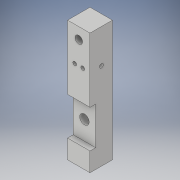
# Autodesk Inventor part: Main Block
Saved by Autodesk Inventor 2018 (Build 220112000, 112)
## iProperties
Created: 2017-09-20
Part Number: Main Block
Material: Generic
Document SubType Name: Modeling
Designer: Intel
Density: 1 g/cm^3
Appearance: Default
Author: Intel
Autodesk Inventor part; units mm, degrees
ref_plane "YZ Plane" through (0, 0, 0) normal (1, 0, 0) x (0, 1, 0)
ref_plane "XZ Plane" through (0, 0, 0) normal (0, 1, 0) x (-1, 0, 0)
ref_plane "XY Plane" through (0, 0, 0) normal (0, 0, 1) x (1, 0, 0)
sketch "Sketch1" plane through (0, 0, 0) normal (0, 0, 1) x (1, 0, 0)
  line L0 (-9.398, 50.8) -> (9.398, 50.8)
  line L1 (9.398, 50.8) -> (9.398, -50.8)
  line L2 (9.398, -50.8) -> (-9.398, -50.8)
  line L3 (-9.398, -50.8) -> (-9.398, 50.8)
  line L4 (-9.398, 50.8) -> (9.398, -50.8) construction
  line L5 (9.398, 50.8) -> (-9.398, -50.8) construction
  point P0 (0, 0)
  dimension "d0" = 18.796
  dimension "d1" = 101.6
  constraints: 12 end point, 2 midpoint, 2 parallel, 1 horizontal, 1 perpendicular
  measures "d0" distance of L1.end L2.end
  measures "d1" distance of L0.end L1.end
extrude "Extrusion1" add sketch "Sketch1" along normal mid plane 18.796
sketch "Sketch2" plane through (0, 0, 9.398) normal (0, 0, 1) x (1, 0, 0)
  line L0 (9.398, -50.8) -> (9.398, 50.8) projected
  line L1 (-9.398, -34.925) -> (9.398, -34.925)
  line L2 (9.398, -34.925) -> (9.398, -3.175)
  line L3 (9.398, -3.175) -> (-9.398, -3.175)
  line L4 (-9.398, -3.175) -> (-9.398, -34.925)
  line L5 (-9.398, -34.925) -> (9.398, -3.175) construction
  line L6 (9.398, -34.925) -> (-9.398, -3.175) construction
  line L7 (-9.398, -50.8) -> (9.398, -50.8) projected
  point P0 (0, 0)
  point P1 (0, -19.05)
  dimension "d4" = 31.75
  dimension "d5" = 15.875
  dimension "d6" = 18.796
  constraints: 12 end point, 2 midpoint, 2 parallel, 1 horizontal, 1 perpendicular, 1 point on line
  measures "d4" distance of L2.end L1.end
  measures "d5" distance between parallel lines of L7 L1
  measures "d6" distance of L2.end L3.end
extrude "Extrusion3" cut sketch "Sketch2" against normal blind 4.7498
sketch "Sketch3" plane through (0, 0, 4.6482) normal (0, 0, 1) x (1, 0, 0)
  circle A0 centre (0, -19.05) radius 3.9624
  line L0 (9.398, -34.925) -> (-9.398, -34.925) projected
  line L1 (9.398, -3.175) -> (9.398, -34.925) projected
  point P0 (0, 0)
  dimension "d11" = 7.9248
  dimension "d12" = 15.875
  dimension "d13" = 9.398
  constraints: 1 centre point
  measures "d11" diameter of A0
  measures "d12" distance from line of L0 A0.centre
  measures "d13" distance from line of L1 A0.centre
extrude "Extrusion4" cut sketch "Sketch3" against normal blind 15.24
sketch "Sketch4" plane through (0, 0, 9.398) normal (0, 0, 1) x (1, 0, 0)
  circle A0 centre (0, 41.275) radius 3.175
  line L0 (9.398, 50.8) -> (-9.398, 50.8) projected
  line L1 (9.398, -3.175) -> (9.398, 50.8) projected
  point P0 (0, 0)
  dimension "d16" = 6.35
  dimension "d17" = 9.525
  dimension "d18" = 9.398
  constraints: 1 centre point
  measures "d16" diameter of A0
  measures "d17" distance from line of L0 A0.centre
  measures "d18" distance from line of L1 A0.centre
extrude "Extrusion5" cut sketch "Sketch4" against normal blind 20.32
sketch "Sketch5" plane through (0, 0, 9.398) normal (0, 0, 1) x (1, 0, 0)
  circle A0 centre (-3.359, 22.225) radius 1.5875
  circle A1 centre (3.359, 22.225) radius 1.5875
  line L0 (9.398, 50.8) -> (-9.398, 50.8) projected
  line L1 (-9.398, 50.8) -> (9.398, 50.8) projected
  line L2 (0, 50.8) -> (0, -50.8) construction
  line L3 (9.398, -50.8) -> (-9.398, -50.8) projected
  circle A2 centre (0, 41.275) radius 3.175 projected
  line L4 (0, 41.275) -> (3.359, 22.225) construction
  line L5 (0, 41.275) -> (-3.359, 22.225) construction
  point P0 (0, 0)
  dimension "d21" = 3.175
  dimension "d22" = 3.175
  dimension "d23" = 28.575
  dimension "d24" = 28.575
  dimension "d25" = 10
  dimension "d26" = 10
  constraints: 6 end point, 2 centre point, 2 midpoint
  measures "d21" diameter of A0
  measures "d22" diameter of A1
  measures "d23" distance from line of L4.end L0
  measures "d24" distance from line of L0 L5.end
  measures "d25" angle of L2 L4
  measures "d26" angle of L5 L2
extrude "Extrusion6" cut sketch "Sketch5" against normal blind 20.32 contours A0
sketch "Sketch6" plane through (0, 0, 9.398) normal (0, 0, 1) x (1, 0, 0)
  circle A0 centre (-3.359, 22.225) radius 1.5875 projected
  circle A1 centre (0, 41.275) radius 3.175 projected
  circle A2 centre (3.359, 22.225) radius 1.5875
  line L0 (0, 41.275) -> (3.359, 22.225) construction
  line L1 (0, 41.275) -> (0, 8.045) construction
  line L2 (9.398, 50.8) -> (-9.398, 50.8) projected
  point P0 (0, 0)
  dimension "d29" = 3.175
  dimension "d31" = 10
  dimension "d32" = 28.575
  constraints: 4 end point, 1 centre point, 1 vertical
  measures "d29" diameter of A2
  measures "d31" angle of L1 L0
  measures "d32" distance from line of L2 L0.end
extrude "Extrusion7" cut sketch "Sketch6" against normal blind 11.0998 contours A2
sketch "Sketch7" plane through (9.398, -50.8, -9.398) normal (1, 0, 0) x (0, 0, -1)
  line L0 (-18.796, 71.4375) -> (-18.796, 74.6125) projected
  circle A0 centre (-9.271, 73.025) radius 1.5875
  line L1 (0, 101.6) -> (0, 0) projected
  line L2 (-18.796, 101.6) -> (0, 101.6) projected
  point P0 (-9.398, 50.8)
  dimension "d35" = 3.175
  dimension "d36" = 9.271
  dimension "d37" = 28.575
  constraints: 1 centre point
  measures "d35" diameter of A0
  measures "d36" distance from line of L1 A0.centre
  measures "d37" distance from line of L2 A0.centre
extrude "Extrusion8" cut sketch "Sketch7" against normal blind 7.62
sketch "Sketch9" plane through (-9.398, -50.8, 9.398) normal (0, -1, 0) x (1, 0, 0)
  point P0 (9.398, -9.398)
  point P1 (9.398, -9.398)
  constraints: 1 coincident
hole "Hole1" at (0, -50.8, 0) direction (0, 1, 0) diameter 6.35 depth 19.05 tip angle 118
thread "Thread1" size "1/4-20 UNC" class "2B" standard "ANSI Unified Screw Threads" full length
equation "\"d24\" = d23"
equation "\"d26\" = d25"
body "Solid1"
